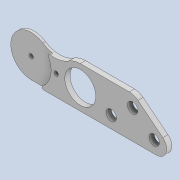
# Autodesk Inventor part: 揺動節
Saved by Autodesk Inventor 2020.4 (Build 244396000, 396)
## iProperties
Created: 2021-05-01
Part Number: 揺動節
Material: 一般
Document SubType Name: Modeling
Designer: happy
Density: 1 g/cm^3
Appearance: 既定
Mass: 5.63716 g
Surface Area: 51.3271 cm^2
Volume: 5.63716 cm^3
Author: happy
Autodesk Inventor part; units mm, degrees
ref_plane "YZ Plane" through (0, 0, 0) normal (1, 0, 0) x (0, 1, 0)
ref_plane "XZ Plane" through (0, 0, 0) normal (0, 1, 0) x (-1, 0, 0)
ref_plane "XY Plane" through (0, 0, 0) normal (0, 0, 1) x (1, 0, 0)
sketch "スケッチ1" plane through (0, 0, 0) normal (0, 0, 1) x (1, 0, 0)
  line L0 (0, 0) -> (30, 0) construction
  line L1 (0, 12) -> (30, 12)
  line L2 (30, -12) -> (0, -12)
  arc A0 (0, 12) -> (0, -12) centre (0, 0) ccw
  arc A1 (30, -12) -> (30, 12) centre (30, 0) ccw
  circle A2 centre (0, 0) radius 1.25
  circle A3 centre (30, 0) radius 9.025
  arc A4 (6.6667, 9.9778) -> (23.3333, 9.9778) centre (15, 22.4499) ccw
  arc A5 (30, 12) -> (30, -12) centre (30, 0) ccw construction
  arc A6 (0, -12) -> (0, 12) centre (0, 0) ccw construction
  arc A7 (6.6667, 9.9778) -> (0, 12) centre (0, 0) ccw
  arc A8 (30, 12) -> (23.3333, 9.9778) centre (30, 0) ccw
  line L3 (30, 12) -> (92.8308, 12)
  line L4 (92.8308, 12) -> (92.8308, -12)
  line L5 (92.8308, -12) -> (30, -12)
  line L6 (30, -12) -> (30, 12)
  circle A9 centre (16, 0) radius 1.25
  dimension "d0" = 30
  dimension "d1" = 12
  dimension "d2" = 2.5
  dimension "d3" = 18.05
  dimension "d6" = 15
  dimension "d11" = 2.5
  dimension "d12" = 16
  constraints: 16 end point, 15 point on circle, 10 centre point, 10 tangent, 3 coincident, 3 parallel, 2 concentric, 2 horizontal, 1 perpendicular, 1 point on line
  measures "d0" distance of L0.start L0.end
  measures "d1" radius of A1
  measures "d2" diameter of A2
  measures "d3" diameter of A3
  measures "d6" radius of A4
  measures "d11" diameter of A9
  measures "d12" distance of A2.centre A9.centre
extrude "押し出し1" add sketch "スケッチ1" along normal blind 3 contours A7 A4 A8 L6 A3 L2 A0 | L3 L4 L5 A1 | A1 L6 A3
sketch "スケッチ2" plane through (0, 0, 3) normal (0, 0, 1) x (1, 0, 0)
  arc A0 (30, 12) -> (23.3333, 9.9778) centre (30, 0) ccw projected
  arc A1 (6.6667, 9.9778) -> (23.3333, 9.9778) centre (15, 22.4499) ccw projected
  arc A2 (6.6667, 9.9778) -> (0, -12) centre (0, 0) ccw projected
  line L0 (0, -12) -> (92.8308, -12) projected
  line L1 (92.8308, -12) -> (92.8308, 12) projected
  line L2 (92.8308, 12) -> (30, 12) projected
  circle A3 centre (0, 0) radius 1.25 projected
  circle A4 centre (30, 0) radius 9.025 projected
  line L3 (0, -12) -> (92.8308, -12) projected
  arc A5 (6.6667, 9.9778) -> (23.3333, 9.9778) centre (15, 22.4499) ccw projected
  arc A6 (0, -12) -> (6.6667, 9.9778) centre (0, 0) ccw
  arc A7 (0, -13) -> (7.8, 10.4) centre (0, 0) ccw
  point P0 (5, -12)
  point P1 (9.9986, 8.3083)
  dimension "d7" = 1
  constraints: 4 point on circle, 2 centre point, 1 concentric
  measures "d7" radial gap between concentric circles of A6 A7
extrude "押し出し2" cut sketch "スケッチ2" against normal blind 1.5 contours A7 L0 A6 A1 | A6 A2
fillet "フィレット1" radius 1 2 edges at (9.9986, 8.3083, 2.25) (5, -12, 2.25)
sketch "スケッチ3" plane through (0, 0, 3) normal (0, 0, 1) x (1, 0, 0)
  arc A0 (30.0122, 16.3221) -> (24.9131, 15.5052) centre (30.0122, 0) ccw
  arc A1 (6.6694, 14.2981) -> (24.9131, 15.5052) centre (15.0061, 26.768) ccw
  arc A2 (6.6694, 14.2981) -> (0, -7.6779) centre (0, 4.3221) ccw
  line L0 (0, -7.6779) -> (30, -7.6779)
  circle A3 centre (0, 0) radius 1.5
  circle A4 centre (16, 0) radius 1.25
  circle A5 centre (48, -5) radius 3.025
  circle A6 centre (73, -5) radius 3.025
  circle A7 centre (60.5, 5) radius 3.025
  line L1 (48, -5) -> (73, -5) construction
  line L2 (61.3547, 12) -> (92.8308, -13.1809)
  line L3 (60.5, 5) -> (73, -5) construction
  line L4 (60.5, 5) -> (60.5, -5) construction
  circle A8 centre (30, 0) radius 9.025 projected
  circle A9 centre (16, 0) radius 1.25 projected
  circle A10 centre (30, 0) radius 9.025 projected
  arc A11 (8.0417, -10.2143) -> (8.6603, -12) centre (8.6603, -11) ccw projected
  line L5 (8.6603, -12) -> (92.8308, -12) projected
  line L6 (92.8308, -12) -> (92.8308, 12) projected
  line L7 (92.8308, 12) -> (30, 12) projected
  arc A12 (30, 12) -> (23.3333, 9.9778) centre (30, 0) ccw projected
  arc A13 (12.4728, 7.6644) -> (23.3333, 9.9778) centre (15, 22.4499) ccw projected
  arc A14 (12.4728, 7.6644) -> (11.4254, 6.2016) centre (12.3043, 6.6787) ccw projected
  arc A15 (8.0417, -10.2143) -> (11.4254, 6.2016) centre (0, 0) ccw projected
  line L8 (92.8308, 12) -> (30, 12) projected
  line L9 (92.8308, -12) -> (92.8308, 12) projected
  point P0 (60.5, 0)
  point P1 (61.3547, 12)
  point P2 (91.3547, -12)
  point P3 (91.3547, -12)
  dimension "d13" = 6.05
  dimension "d14" = 6.05
  dimension "d15" = 6.05
  dimension "d16" = 25
  dimension "d17" = 10
  dimension "d19" = 6
  dimension "d20" = 18
  constraints: 10 end point, 8 centre point, 6 point on circle, 2 horizontal alignment, 2 midpoint, 2 point on line, 1 horizontal, 1 parallel, 1 vertical, 1 vertical alignment
  measures "d13" diameter of A5
  measures "d14" diameter of A6
  measures "d15" diameter of A7
  measures "d16" distance of L1.end L1.start
  measures "d17" vertical distance of L3.start L1.start
  measures "d19" distance between parallel lines of L2 L3
  measures "d20" horizontal distance of A8.centre L1.start
extrude "押し出し3" cut sketch "スケッチ3" against normal blind 10 contours A5 | A6 | A7 | L7 L6 L5 L2
fillet "フィレット2" radius 8 1 edges at (61.3547, 12, 1.5)
fillet "フィレット3" radius 6 1 edges at (91.3547, -12, 1.5)
